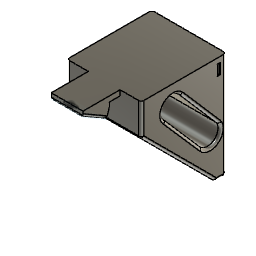
armazon de dispositivo de reconocimiento facial v1 (Autodesk Fusion 360 design; units mm, degrees)
Autodesk Fusion 360 part; units mm, degrees
note: some values were not read from the file. Set by a fixed rule: which sketch regions a step uses.
sketch "Boceto1" plane through (0, 0, 0) normal (0, 1, 0) x (1, 0, 0)
  line L0 (0, -200) -> (70, -200)
  line L1 (0, -200) -> (-70, -200)
  line L2 (-70, -200) -> (-70, 0)
  line L3 (-70, 0) -> (70, 0)
  line L4 (70, 0) -> (70, -200)
  dimension "d1" = 200
  dimension "d2" = 70
  dimension "d3" = 70
  constraint perpendicular L1 L2
  constraint perpendicular L0 L4
  measures "d1" distance of origin L0.start
  measures "d2" distance of L0.start L0.end
  measures "d3" distance of L0.start L1.end
extrude "Extruir1" add sketch "Boceto1" along normal blind 160
sketch "Boceto2" plane through (70, 0, 0) normal (1, 0, 0) x (0, 1, 0)
  line L0 (0, 200) -> (0, 0)
  line L1 (0, 0) -> (160, 0)
  line L2 (160, 0) -> (160, 200)
  line L3 (160, 200) -> (0, 200)
  line L4 (140, 0) -> (0, 140)
  line L5 (430, 170) -> (420, 170)
  constraint coincident L1 L4.start
  constraint coincident L0 L4.end
  constraint perpendicular L2 L5
extrude "Extruir2" cut sketch "Boceto2" against normal blind 140 contours L0 L1 L4
sketch "Boceto3" plane through (0, 0, 0) normal (0, -1, 0) x (1, 0, 0)
  line L0 (-70, 140) -> (70, 140)
  line L1 (70, 140) -> (70, 200)
  line L2 (70, 200) -> (-70, 200)
  line L3 (-70, 200) -> (-70, 140)
  line L4 (30, 200) -> (30, 190)
  line L5 (30, 190) -> (-30, 190)
  line L6 (-30, 190) -> (-30, 200)
  constraint coincident L2 L4.start
  constraint perpendicular L2 L4
  constraint perpendicular L4 L5
  constraint coincident L2 L6.end
  constraint perpendicular L2 L6
extrude "Extruir3" add sketch "Boceto3" along normal blind 70 contours L2 L4 L5 L6
sketch "Boceto4" plane through (0, 0, 190) normal (0, 0, -1) x (1, 0, 0)
  line L0 (-30, 0) -> (30, 0)
  line L1 (30, 0) -> (30, 70)
  line L2 (30, 70) -> (-30, 70)
  line L3 (-30, 70) -> (-30, 0)
  line L4 (-30, 20) -> (30, 20)
  constraint coincident L3 L4.start
  constraint coincident L1 L4.end
  constraint perpendicular L1 L4
revolve "Revolución1" add sketch "Boceto4" angle 30 about axis through (30, -70, 190) along (-1, 0, 0) contours L1 L2 L3 L4
sketch "Boceto5" plane through (0, 64.7724, 112.1891) normal (0, -0.5, -0.866025) x (1, 0, 0)
  line L0 (-30, 105.6218) -> (30, 105.6218)
  line L1 (30, 105.6218) -> (30, 155.6218)
  line L2 (30, 155.6218) -> (-30, 155.6218)
  line L3 (-30, 155.6218) -> (-30, 105.6218)
  circle A0 centre (-15, 130) radius 10
  circle A1 centre (-15, 130) radius 7.5
  dimension "d11" = 15
  constraint concentric A0 A1
  measures "d11" diameter of A1
extrude "Extruir4" cut sketch "Boceto5" against normal blind 5 contours A1
sketch "Boceto6" plane through (0, 64.7724, 112.1891) normal (0, -0.5, -0.866025) x (1, 0, 0)
  circle A0 centre (-15, 130) radius 7.5
  line L0 (-30, 105.6218) -> (30, 105.6218)
  line L1 (30, 105.6218) -> (30, 155.6218)
  line L2 (30, 155.6218) -> (-30, 155.6218)
  line L3 (-30, 155.6218) -> (-30, 105.6218)
  circle A1 centre (-15, 130) radius 10
  dimension "d14" = 20
  constraint concentric A0 A1
  measures "d14" diameter of A1
sketch "Boceto7" plane through (70, 0, 0) normal (1, 0, 0) x (0, 1, 0)
  line L0 (0, 140) -> (140, 0)
  line L1 (140, 0) -> (160, 0)
  line L2 (160, 0) -> (160, 200)
  line L3 (160, 200) -> (0, 200)
  line L4 (0, 200) -> (0, 140)
  line L5 (0, 140) -> (0, 160)
  line L6 (0, 160) -> (160, 0)
  circle A0 centre (130, 80) radius 20
  circle A1 centre (60, 160) radius 20
  line L7 (45.8852, 145.8306) -> (114.9426, 66.8366)
  line L8 (147.3803, 89.8957) -> (75.0996, 173.1149)
  dimension "d15" = 20
  constraint coincident L0.start L4.end
  constraint parallel L4 L5
  constraint coincident L1.end L2.start
  constraint coincident A1 L7.start
  constraint coincident A0 L7.end
  constraint tangent A0 L7
  constraint coincident A0 L8.start
  constraint coincident A1 L8.end
  constraint tangent A1 L8
  measures "d15" distance of L0.start L5.end
extrude "Extruir5" cut sketch "Boceto7" against normal blind 170 contours A0 L8 | A0 A1 L7 L8 | A1 picked at (118.5803, 82.9284)
sketch "Boceto8" plane through (0, 70, 70) normal (0, -0.707107, -0.707107) x (1, 0, 0)
  line L0 (70, -98.9949) -> (70, 98.9949)
  line L1 (70, 98.9949) -> (-70, 98.9949)
  line L2 (-70, 98.9949) -> (-70, -98.9949)
  line L3 (-70, -98.9949) -> (70, -98.9949)
  line L4 (-60, 90) -> (60, 90)
  line L5 (60, 90) -> (60, -90)
  line L6 (-60, 90) -> (-60, -90)
  line L7 (-60, -90) -> (60, -90)
  constraint perpendicular L0 L4
  constraint perpendicular L4 L5
  constraint perpendicular L3 L6
  constraint perpendicular L5 L7
extrude "Extruir6" cut sketch "Boceto8" against normal blind 15 contours L4 L5 L6 L7
sketch "Boceto9" plane through (70, 0, 0) normal (1, 0, 0) x (0, 1, 0)
  arc A0 (75.0996, 173.1149) -> (45.8852, 145.8306) centre (60, 160) ccw
  line L0 (75.0996, 173.1149) -> (147.3803, 89.8957)
  arc A1 (114.9426, 66.8366) -> (147.3803, 89.8957) centre (130, 80) ccw
  line L1 (114.9426, 66.8366) -> (45.8852, 145.8306)
  line L2 (0, 140) -> (140, 0)
  line L3 (140, 0) -> (160, 0)
  line L4 (160, 0) -> (160, 200)
  line L5 (160, 200) -> (0, 200)
  line L6 (0, 200) -> (0, 140)
  line L7 (140, 190) -> (150, 190)
  line L8 (150, 190) -> (150, 170)
  line L9 (150, 170) -> (140, 170)
  line L10 (147, 171) -> (147, 189)
  line L11 (147, 189) -> (149, 189)
  line L12 (149, 189) -> (149, 171)
  line L13 (149, 171) -> (147, 171)
  line L14 (143.8463, 170) -> (143.8463, 190)
  dimension "d20" = 20
  constraint perpendicular L7 L8
  constraint perpendicular L9 L10
  constraint perpendicular L10 L11
  constraint perpendicular L9 L12
  constraint perpendicular L10 L13
  constraint coincident L9 L14.start
  constraint coincident L7 L14.end
  constraint perpendicular L7 L14
  measures "d20" distance of L7.end L8.end
extrude "Extruir7" cut sketch "Boceto9" against normal blind 15 contours L7 L8 L9 L14
fillet "Empalme1" radius 5 19 edges at (70, 0, 170) (70, 70, 70) (70, 150, 0) (70, 160, 100) (-70, 0, 170) (-70, 70, 70) (-70, 150, 0) (-70, 160, 100) (-70, 80.4139, 106.3336) (-70, 141.5879, 63.6991) (-70, 111.24, 131.5053) (-70, 46.349, 174.6167) (70, 141.5879, 63.6991) (70, 80.4139, 106.3336) (70, 46.349, 174.6167) (70, 111.24, 131.5053) (0, 160, 0) (0, 140, 0) (0, 0, 140)
fillet "Empalme2" radius 5 4 edges at (30, -48.3494, 177.5) (0, -26.6987, 165) (-30, -48.3494, 177.5) (0, -70, 190)
